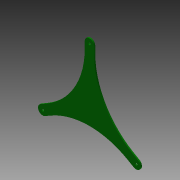
# Autodesk Inventor part: Light Sensor PCB
Saved by Autodesk Inventor 2015 (Build 190159000, 159)
## iProperties
Created: 2016-02-18
Part Number: Light Sensor PCB
Material: Generic
Document SubType Name: Modeling
Designer: 23902
Density: 1 g/cm^3
Appearance: Default
Author: 23902
Autodesk Inventor part; units mm, degrees
ref_plane "YZ Plane" through (0, 0, 0) normal (1, 0, 0) x (0, 1, 0)
ref_plane "XZ Plane" through (0, 0, 0) normal (0, 1, 0) x (-1, 0, 0)
ref_plane "XY Plane" through (0, 0, 0) normal (0, 0, 1) x (1, 0, 0)
sketch "Sketch1" plane through (0, 0, 0) normal (0, 1, 0) x (-1, 0, 0)
  circle A0 centre (-63.396, -33.6837) radius 1.6
  line L0 (-66.396, -28.4875) -> (-58.7743, -24.0871)
  line L1 (-60.396, -38.8798) -> (-52.7743, -34.4794)
  line L2 (-59.0659, -31.1837) -> (-59.9409, -29.6682)
  line L3 (-59.0659, -31.1837) -> (-58.1909, -32.6992)
  line L4 (-59.9409, -29.6682) -> (-58.2089, -28.6682)
  line L5 (-58.2089, -28.6682) -> (-56.4589, -31.6992)
  line L6 (-56.4589, -31.6992) -> (-58.1909, -32.6992)
  line L7 (-56.4678, -29.6837) -> (-57.3428, -28.1682)
  line L8 (-56.4678, -29.6837) -> (-55.5928, -31.1992)
  line L9 (-57.3428, -28.1682) -> (-55.6108, -27.1682)
  line L10 (-55.6108, -27.1682) -> (-53.8608, -30.1992)
  line L11 (-53.8608, -30.1992) -> (-55.5928, -31.1992)
  line L12 (-48.5004, -25.0837) -> (-49.3754, -23.5682)
  line L13 (-48.5004, -25.0837) -> (-47.6254, -26.5992)
  line L14 (-49.3754, -23.5682) -> (-47.6433, -22.5682)
  line L15 (-47.6433, -22.5682) -> (-45.8933, -25.5992)
  line L16 (-45.8933, -25.5992) -> (-47.6254, -26.5992)
  line L17 (-45.9023, -23.5837) -> (-46.7773, -22.0682)
  line L18 (-45.9023, -23.5837) -> (-45.0273, -25.0992)
  line L19 (-46.7773, -22.0682) -> (-45.0453, -21.0682)
  line L20 (-45.0453, -21.0682) -> (-43.2953, -24.0992)
  line L21 (-43.2953, -24.0992) -> (-45.0273, -25.0992)
  line L22 (-37.9349, -18.9837) -> (-38.8099, -17.4682)
  line L23 (-37.9349, -18.9837) -> (-37.0599, -20.4992)
  line L24 (-38.8099, -17.4682) -> (-37.0778, -16.4682)
  line L25 (-37.0778, -16.4682) -> (-35.3278, -19.4992)
  line L26 (-35.3278, -19.4992) -> (-37.0599, -20.4992)
  line L27 (-35.3368, -17.4837) -> (-36.2118, -15.9682)
  line L28 (-35.3368, -17.4837) -> (-34.4618, -18.9992)
  line L29 (-36.2118, -15.9682) -> (-34.4798, -14.9682)
  line L30 (-34.4798, -14.9682) -> (-32.7298, -17.9992)
  line L31 (-32.7298, -17.9992) -> (-34.4618, -18.9992)
  line L32 (-27.3694, -12.8837) -> (-28.2444, -11.3682)
  line L33 (-27.3694, -12.8837) -> (-26.4944, -14.3992)
  line L34 (-28.2444, -11.3682) -> (-26.5123, -10.3682)
  line L35 (-26.5123, -10.3682) -> (-24.7623, -13.3992)
  line L36 (-24.7623, -13.3992) -> (-26.4944, -14.3992)
  line L37 (-24.7713, -11.3837) -> (-25.6463, -9.8682)
  line L38 (-24.7713, -11.3837) -> (-23.8963, -12.8992)
  line L39 (-25.6463, -9.8682) -> (-23.9143, -8.8682)
  line L40 (-23.9143, -8.8682) -> (-22.1643, -11.8992)
  line L41 (-22.1643, -11.8992) -> (-23.8963, -12.8992)
  circle A1 centre (57.8475, -33.6837) radius 1.6
  line L42 (54.8475, -38.8798) -> (47.2257, -34.4794)
  line L43 (60.8475, -28.4875) -> (53.2257, -24.0871)
  line L44 (53.5174, -31.1837) -> (52.6424, -32.6992)
  line L45 (53.5174, -31.1837) -> (54.3924, -29.6682)
  line L46 (52.6424, -32.6992) -> (50.9103, -31.6992)
  line L47 (50.9103, -31.6992) -> (52.6603, -28.6682)
  line L48 (52.6603, -28.6682) -> (54.3924, -29.6682)
  line L49 (50.9193, -29.6837) -> (50.0443, -31.1992)
  line L50 (50.9193, -29.6837) -> (51.7943, -28.1682)
  line L51 (50.0443, -31.1992) -> (48.3123, -30.1992)
  line L52 (48.3123, -30.1992) -> (50.0623, -27.1682)
  line L53 (50.0623, -27.1682) -> (51.7943, -28.1682)
  line L54 (42.9519, -25.0837) -> (42.0769, -26.5992)
  line L55 (42.9519, -25.0837) -> (43.8269, -23.5682)
  line L56 (42.0769, -26.5992) -> (40.3448, -25.5992)
  line L57 (40.3448, -25.5992) -> (42.0948, -22.5682)
  line L58 (42.0948, -22.5682) -> (43.8269, -23.5682)
  line L59 (40.3538, -23.5837) -> (39.4788, -25.0992)
  line L60 (40.3538, -23.5837) -> (41.2288, -22.0682)
  line L61 (39.4788, -25.0992) -> (37.7468, -24.0992)
  line L62 (37.7468, -24.0992) -> (39.4968, -21.0682)
  line L63 (39.4968, -21.0682) -> (41.2288, -22.0682)
  line L64 (32.3864, -18.9837) -> (31.5114, -20.4992)
  line L65 (32.3864, -18.9837) -> (33.2614, -17.4682)
  line L66 (31.5114, -20.4992) -> (29.7793, -19.4992)
  line L67 (29.7793, -19.4992) -> (31.5293, -16.4682)
  line L68 (31.5293, -16.4682) -> (33.2614, -17.4682)
  line L69 (29.7883, -17.4837) -> (28.9133, -18.9992)
  line L70 (29.7883, -17.4837) -> (30.6633, -15.9682)
  line L71 (28.9133, -18.9992) -> (27.1812, -17.9992)
  line L72 (27.1812, -17.9992) -> (28.9312, -14.9682)
  line L73 (28.9312, -14.9682) -> (30.6633, -15.9682)
  line L74 (21.8209, -12.8837) -> (20.9459, -14.3992)
  line L75 (21.8209, -12.8837) -> (22.6959, -11.3682)
  line L76 (20.9459, -14.3992) -> (19.2138, -13.3992)
  line L77 (19.2138, -13.3992) -> (20.9638, -10.3682)
  line L78 (20.9638, -10.3682) -> (22.6959, -11.3682)
  line L79 (19.2228, -11.3837) -> (18.3478, -12.8992)
  line L80 (19.2228, -11.3837) -> (20.0978, -9.8682)
  line L81 (18.3478, -12.8992) -> (16.6157, -11.8992)
  line L82 (16.6157, -11.8992) -> (18.3657, -8.8682)
  line L83 (18.3657, -8.8682) -> (20.0978, -9.8682)
  circle A2 centre (-2.7743, 71.3163) radius 1.6
  line L84 (3.2257, 71.3163) -> (3.2257, 62.5154)
  line L85 (-8.7743, 71.3163) -> (-8.7743, 62.5154)
  line L86 (-2.7743, 66.3163) -> (-1.0243, 66.3163)
  line L87 (-2.7743, 66.3163) -> (-4.5243, 66.3163)
  line L88 (-1.0243, 66.3163) -> (-1.0243, 64.3163)
  line L89 (-1.0243, 64.3163) -> (-4.5243, 64.3163)
  line L90 (-4.5243, 64.3163) -> (-4.5243, 66.3163)
  line L91 (-2.7743, 63.3163) -> (-1.0243, 63.3163)
  line L92 (-2.7743, 63.3163) -> (-4.5243, 63.3163)
  line L93 (-1.0243, 63.3163) -> (-1.0243, 61.3163)
  line L94 (-1.0243, 61.3163) -> (-4.5243, 61.3163)
  line L95 (-4.5243, 61.3163) -> (-4.5243, 63.3163)
  line L96 (-2.7743, 54.1163) -> (-1.0243, 54.1163)
  line L97 (-2.7743, 54.1163) -> (-4.5243, 54.1163)
  line L98 (-1.0243, 54.1163) -> (-1.0243, 52.1163)
  line L99 (-1.0243, 52.1163) -> (-4.5243, 52.1163)
  line L100 (-4.5243, 52.1163) -> (-4.5243, 54.1163)
  line L101 (-2.7743, 51.1163) -> (-1.0243, 51.1163)
  line L102 (-2.7743, 51.1163) -> (-4.5243, 51.1163)
  line L103 (-1.0243, 51.1163) -> (-1.0243, 49.1163)
  line L104 (-1.0243, 49.1163) -> (-4.5243, 49.1163)
  line L105 (-4.5243, 49.1163) -> (-4.5243, 51.1163)
  line L106 (-2.7743, 41.9163) -> (-1.0243, 41.9163)
  line L107 (-2.7743, 41.9163) -> (-4.5243, 41.9163)
  line L108 (-1.0243, 41.9163) -> (-1.0243, 39.9163)
  line L109 (-1.0243, 39.9163) -> (-4.5243, 39.9163)
  line L110 (-4.5243, 39.9163) -> (-4.5243, 41.9163)
  line L111 (-2.7743, 38.9163) -> (-1.0243, 38.9163)
  line L112 (-2.7743, 38.9163) -> (-4.5243, 38.9163)
  line L113 (-1.0243, 38.9163) -> (-1.0243, 36.9163)
  line L114 (-1.0243, 36.9163) -> (-4.5243, 36.9163)
  line L115 (-4.5243, 36.9163) -> (-4.5243, 38.9163)
  line L116 (-2.7743, 29.7163) -> (-1.0243, 29.7163)
  line L117 (-2.7743, 29.7163) -> (-4.5243, 29.7163)
  line L118 (-1.0243, 29.7163) -> (-1.0243, 27.7163)
  line L119 (-1.0243, 27.7163) -> (-4.5243, 27.7163)
  line L120 (-4.5243, 27.7163) -> (-4.5243, 29.7163)
  line L121 (-2.7743, 26.7163) -> (-1.0243, 26.7163)
  line L122 (-2.7743, 26.7163) -> (-4.5243, 26.7163)
  line L123 (-1.0243, 26.7163) -> (-1.0243, 24.7163)
  line L124 (-1.0243, 24.7163) -> (-4.5243, 24.7163)
  line L125 (-4.5243, 24.7163) -> (-4.5243, 26.7163)
  arc A3 (3.2257, 71.3163) -> (-8.7743, 71.3163) centre (-2.7743, 71.3163) ccw
  arc A4 (-66.396, -28.4875) -> (-60.396, -38.8798) centre (-63.396, -33.6837) ccw
  arc A5 (54.8475, -38.8798) -> (60.8475, -28.4875) centre (57.8475, -33.6837) ccw
  arc A6 (-58.7743, -24.0871) -> (-8.7743, 62.5154) centre (-108.7743, 62.5154) ccw
  arc A7 (3.2257, 62.5154) -> (53.2257, -24.0871) centre (103.2257, 62.5154) ccw
  arc A8 (47.2257, -34.4794) -> (-52.7743, -34.4794) centre (-2.7743, -121.082) ccw
  point P0 (0, 0)
  constraints: 252 end point, 12 point on circle, 9 centre point
extrude "Extrusion1" add sketch "Sketch1" along normal blind 1.6 contours L0 A6 L85 A3 L84 A7 L43 A5 L42 A8 L1 A4 | L2 L4 L5 L6 L3 | L7 L9 L10 L11 L8 | L12 L14 L15 L16 L13 | L17 L19 L20 L21 L18 | L22 L24 L25 L26 L23 | L27 L29 L30 L31 L28 | L32 L34 L35 L36 L33 | L37 L39 L40 L41 L38 | L44 L46 L47 L48 L45 | L49 L51 L52 L53 L50 | L54 L56 L57 L58 L55 | L59 L61 L62 L63 L60 | L64 L66 L67 L68 L65 | L69 L71 L72 L73 L70 | L74 L76 L77 L78 L75 | L79 L81 L82 L83 L80 | L86 L88 L89 L90 L87 | L91 L93 L94 L95 L92 | L96 L98 L99 L100 L97 | L101 L103 L104 L105 L102 | L106 L108 L109 L110 L107 | L111 L113 L114 L115 L112 | L116 L118 L119 L120 L117 | L121 L123 L124 L125 L122
body "Solid1"
